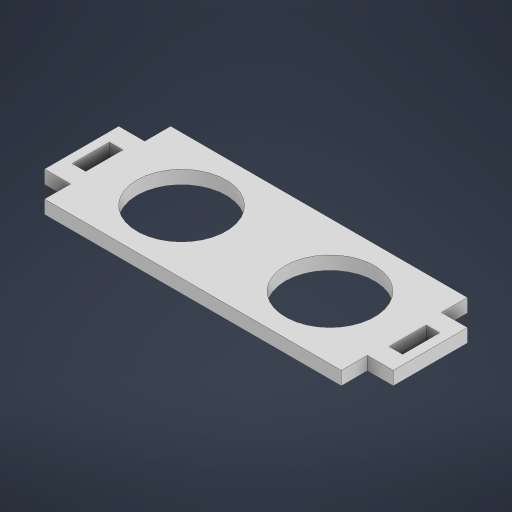
# Autodesk Inventor part: APM_001-2
Saved by Autodesk Inventor 2024 (Build 280153000, 153)
## iProperties
Created: 2023-05-12
Part Number: APM_001-2
Material: Genérico
Document SubType Name: Modeling
Designer: javie
Density: 1 g/cm^3
Appearance: Valor por defecto
Author: javie
Autodesk Inventor part; units mm, degrees
ref_plane "YZ Plane" through (0, 0, 0) normal (1, 0, 0) x (0, 1, 0)
ref_plane "XZ Plane" through (0, 0, 0) normal (0, 1, 0) x (-1, 0, 0)
ref_plane "XY Plane" through (0, 0, 0) normal (0, 0, 1) x (1, 0, 0)
sketch "Boceto1" plane through (0, 0, 0) normal (0, 1, 0) x (-1, 0, 0)
  line L0 (200, 169.7039) -> (-200, 169.7039)
  line L1 (-235, 134.7039) -> (-235, 34.7039)
  line L2 (-200, -0.2961) -> (200, -0.2961)
  line L3 (235, 34.7039) -> (235, 134.7039)
  circle A0 centre (100, 85) radius 60
  line L4 (222.5, 109.7039) -> (204.5, 109.7039)
  line L5 (204.5, 109.7039) -> (204.5, 59.7039)
  line L6 (204.5, 59.7039) -> (222.5, 59.7039)
  line L7 (222.5, 59.7039) -> (222.5, 109.7039)
  line L8 (235, 134.7039) -> (200, 134.7039)
  line L9 (200, 134.7039) -> (200, 169.7039)
  line L10 (235, 34.7039) -> (200, 34.7039)
  line L11 (200, 34.7039) -> (200, -0.2961)
  line L12 (-235, 34.7039) -> (-235, 134.7039)
  circle A1 centre (-100, 85) radius 60
  line L13 (-222.5, 109.7039) -> (-204.5, 109.7039)
  line L14 (-204.5, 109.7039) -> (-204.5, 59.7039)
  line L15 (-204.5, 59.7039) -> (-222.5, 59.7039)
  line L16 (-222.5, 59.7039) -> (-222.5, 109.7039)
  line L17 (-235, 134.7039) -> (-200, 134.7039)
  line L18 (-200, 134.7039) -> (-200, 169.7039)
  line L19 (-235, 34.7039) -> (-200, 34.7039)
  line L20 (-200, 34.7039) -> (-200, -0.2961)
  point P0 (0, 0)
  point P1 (235, 84.7039)
  point P2 (217.5, 134.7039)
  point P3 (-235, 84.7039)
  point P4 (-217.5, 134.7039)
  dimension "d4" = 120
  dimension "d5" = 18
  dimension "d6" = 35
  dimension "d7" = 35
  dimension "d8" = 35
  dimension "d9" = 50
  dimension "d10" = 25
  dimension "d11" = 12.5
  dimension "d12" = 100
  dimension "d15" = 470
  dimension "d16" = 12.5
  dimension "d17" = 18
  constraints: 42 end point, 4 parallel, 4 perpendicular, 4 point on line, 3 horizontal, 3 midpoint, 2 centre point
  measures "d4" diameter of A0
  measures "d5" distance of L6.end L5.end
  measures "d6" distance of L3.end L8.end
  measures "d7" distance of L0.start L8.end
  measures "d8" distance of L2.end L10.end
  measures "d9" distance of L4.end L5.end
  measures "d10" vertical distance of point (217.5, 134.704) L4.start
  measures "d11" distance between parallel lines of L3 L7
  measures "d12" distance from line of A0.centre L11
  measures "d15" distance between parallel lines of L1 L3
  measures "d16" distance between parallel lines of L1 L16
  measures "d17" distance between parallel lines of L16 L14
extrude "Extrusión1" add sketch "Boceto1" along normal blind 18
